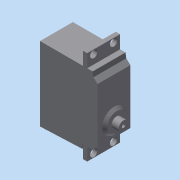
# Autodesk Inventor part: Servo
Saved by Autodesk Inventor 2017 (Build 210142000, 142)
## iProperties
Created: 2014-01-17
Part Number: Servo
Material: Generic
Document SubType Name: Modeling
Designer: Derek
Density: 1 g/cm^3
Appearance: Default
Author: Derek
Autodesk Inventor part; units mm, degrees
ref_plane "YZ Plane" through (0, 0, 0) normal (1, 0, 0) x (0, 1, 0)
ref_plane "XZ Plane" through (0, 0, 0) normal (0, 1, 0) x (-1, 0, 0)
ref_plane "XY Plane" through (0, 0, 0) normal (0, 0, 1) x (1, 0, 0)
sketch "Sketch1" plane through (0, 0, 0) normal (0, 0, 1) x (1, 0, 0)
  line L0 (-13.4156, 8.7484) -> (-13.4156, -32.0313)
  line L1 (-13.4156, -32.0313) -> (12.4924, -32.0313)
  line L2 (-13.4156, 8.7484) -> (12.4924, 8.7484)
  line L3 (12.4924, -32.0313) -> (12.4924, -39.9307)
  line L4 (12.4924, -39.9307) -> (15.0324, -39.9307)
  line L5 (15.0324, -39.9307) -> (15.0324, -32.0313)
  line L6 (12.4924, 8.7484) -> (12.4924, 16.6478)
  line L7 (12.4924, 16.6478) -> (15.0324, 16.6478)
  line L8 (15.0324, 16.6478) -> (15.0324, 8.7484)
  line L9 (15.0324, 8.7484) -> (18.3344, 8.7484)
  line L10 (18.3344, 8.7484) -> (18.3344, -8.4728)
  line L11 (18.3344, -8.4728) -> (20.8744, -8.4728)
  line L12 (20.8744, -8.4728) -> (18.3344, 8.7484)
  line L13 (20.8744, -8.4728) -> (20.8744, -28.5642)
  line L14 (15.0324, -32.0313) -> (18.3344, -32.0313)
  line L15 (18.3344, -32.0313) -> (20.8744, -28.5642)
  line L16 (20.8744, -28.5642) -> (21.3189, -28.5642)
  line L17 (21.3189, -28.5642) -> (21.3189, -29.1611)
  line L18 (21.3189, -29.1611) -> (18.6698, -31.5735)
  line L19 (21.3189, -28.5642) -> (21.3189, 3.6684)
  line L20 (18.3344, 8.7484) -> (18.3344, 5.8274)
  line L21 (18.3344, 5.8274) -> (18.7561, 5.8896)
  line L22 (21.3189, 3.6684) -> (18.7561, 5.8896)
  point P0 (0, 0)
  dimension "d0" = 40.7797
  dimension "d1" = 25.908
  dimension "d2" = 7.8994
  dimension "d3" = 2.54
  dimension "d4" = 7.8994
  dimension "d5" = 3.302
  dimension "d6" = 17.2212
  dimension "d7" = 2.54
  dimension "d8" = 20.0914
  dimension "d9" = 0.4445
  dimension "d10" = 0.5969
  dimension "d11" = 5.08
  dimension "d12" = 2.921
  constraints: 46 end point, 12 perpendicular, 4 parallel, 4 point on line, 1 collinear, 1 vertical
  measures "d0" distance of L0.start L0.end
  measures "d1" distance of L0.end L1.end
  measures "d2" distance of L1.end L3.end
  measures "d3" distance of L3.end L4.end
  measures "d4" distance of L2.end L6.end
  measures "d5" distance of L8.end L9.end
  measures "d6" distance of L9.end L10.end
  measures "d7" distance of L10.end L11.end
  measures "d8" distance of L11.end L13.end
  measures "d9" distance of L13.end L16.end
  measures "d10" distance of L16.end L17.end
  measures "d11" distance from line of L19.end L9
  measures "d12" distance of L9.end L20.end
extrude "Extrusion1" add sketch "Sketch1" along normal blind 19.812
sketch "Sketch2" plane through (21.3189, -29.1611, 0) normal (1, 0, 0) x (0, 0, -1)
  line L0 (-19.812, 0) -> (-19.812, 32.8295) projected
  line L1 (0, 0) -> (-19.812, 0) projected
  line L2 (-9.906, 0) -> (-9.906, 1.5621)
  line L3 (-19.812, 0) -> (-19.812, 8.8138)
  line L4 (-19.812, 8.8138) -> (-9.906, 8.8138)
  line L5 (-9.906, 8.8138) -> (-9.906, 1.5621)
  circle A0 centre (-9.906, 8.8138) radius 7.2517
  line L6 (-2.6543, 8.8138) -> (-4.2037, 8.8138)
  circle A1 centre (-9.906, 8.8138) radius 5.7023
  point P0 (0, 29.1611)
  dimension "d15" = 1.5621
  dimension "d16" = 8.8138
  dimension "d17" = 1.5494
  constraints: 10 end point, 3 perpendicular, 2 coincident, 2 point on circle, 2 point on line, 1 centre point, 1 horizontal alignment, 1 midpoint, 1 parallel, 2 other
  measures "d15" distance of L2.start L2.end
  measures "d16" distance of L0.start L3.end
  measures "d17" distance of L6.start L6.end
extrude "Extrusion2" add sketch "Sketch2" along normal blind 1.524 contours A0 L6 A1 L4 | L4 A1 L5 A0 | L5 A1 L6 A0 | A1 L5 L4 | L4 L5 A1
chamfer "Chamfer1" distance 1.5748 distance2 1.524 1 edges at (22.8429, -13.0956, 9.906) measured on face at (22.8429, -13.5956, 9.906)
sketch "Sketch3" plane through (22.8429, -20.3473, 9.906) normal (1, 0, 0) x (0, 0, -1)
  circle A0 centre (0, 0) radius 5.6769 projected
  circle A1 centre (0, 0) radius 2.9909
  point P0 (9.906, 20.3473)
  dimension "d23" = 5.9817
  constraints: 1 centre point, 1 coincident
  measures "d23" diameter of A1
extrude "Extrusion3" add sketch "Sketch3" along normal blind 4.2164 contours A1
sketch "Sketch4" plane through (27.0593, -20.3473, 9.906) normal (1, 0, 0) x (0, 0, -1)
  circle A0 centre (0, 0) radius 2.9909 projected
  circle A1 centre (0, 0) radius 1.016
  point P0 (9.906, 20.3473)
  dimension "d26" = 2.032
  constraints: 1 centre point, 1 coincident
  measures "d26" diameter of A1
extrude "Extrusion4" cut sketch "Sketch4" against normal blind 4.2164 contours A1
sketch "Sketch5" plane through (15.0324, 8.7484, 0) normal (1, 0, 0) x (0, 0, -1)
  line L0 (0, 0) -> (0, 7.8994) projected
  line L1 (0, 7.8994) -> (-19.812, 7.8994) projected
  line L2 (-19.812, 0) -> (-19.812, 7.8994) projected
  circle A0 centre (-3.9116, 5.461) radius 2.159
  circle A1 centre (-15.9004, 5.461) radius 2.159
  line L3 (-19.812, -48.6791) -> (-19.812, -40.7797) projected
  line L4 (0, -48.6791) -> (-19.812, -48.6791) projected
  line L5 (0, -48.6791) -> (0, -40.7797) projected
  circle A2 centre (-15.9004, -46.2407) radius 2.159
  circle A3 centre (-3.9116, -46.2407) radius 2.159
  point P0 (0, -8.7484)
  dimension "d29" = 4.318
  dimension "d30" = 4.318
  dimension "d31" = 2.4384
  dimension "d32" = 2.4384
  dimension "d33" = 3.9116
  dimension "d34" = 3.9116
  dimension "d35" = 2.4384
  dimension "d36" = 2.4384
  constraints: 4 centre point
  measures "d29" diameter of A0
  measures "d30" diameter of A1
  measures "d31" distance from line of A0.centre L1
  measures "d32" distance from line of L1 A1.centre
  measures "d33" distance from line of A1.centre L2
  measures "d34" distance from line of A0.centre L0
  measures "d35" distance from line of L4 A2.centre
  measures "d36" distance from line of L4 A3.centre
extrude "Extrusion5" cut sketch "Sketch5" against normal through all
sketch "Sketch6" plane through (-13.4156, -32.0313, 0) normal (0, -1, 0) x (1, 0, 0)
  line L0 (0, 0) -> (25.908, 0) projected
  line L1 (0, 19.812) -> (25.908, 19.812) projected
  line L2 (0, 19.812) -> (0, 0)
  line L3 (0, 19.812) -> (25.4, 19.812)
  line L4 (25.4, 19.812) -> (25.4, 0)
  line L5 (25.4, 0) -> (0, 0)
  point P0 (13.4156, 0)
  dimension "d39" = 25.4
  constraints: 8 end point, 2 perpendicular, 2 point on line, 1 collinear
  measures "d39" distance of L1.start L3.end
extrude "Extrusion6" add sketch "Sketch6" along normal blind 3.81
sketch "Sketch7" plane through (0, 0, 0) normal (0, 0, -1) x (-1, 0, 0)
  line L0 (-11.9844, -32.0313) -> (-11.9844, -35.8413) projected
  line L1 (13.4156, -35.8413) -> (-11.9844, -35.8413) projected
  line L2 (-11.9844, -32.0313) -> (-11.9844, -34.7745)
  line L3 (-11.9844, -34.7745) -> (13.4156, -35.8413)
  line L4 (13.4156, -35.8413) -> (-11.9844, -35.8413)
  line L5 (-11.9844, -35.8413) -> (-11.9844, -34.7745)
  point P0 (0, 0)
  dimension "d42" = 2.7432
  constraints: 8 end point, 2 collinear, 1 point on line
  measures "d42" distance of L0.start L2.end
extrude "Extrusion7" cut sketch "Sketch7" against normal through all
body "Solid1"
